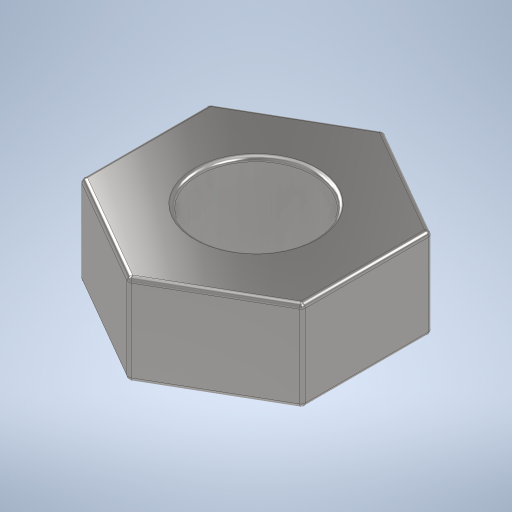
# Autodesk Inventor part: Threaded Rod Nut
Saved by Autodesk Inventor 2024 (Build 280153000, 153)
## iProperties
Created: 2023-12-05
Part Number: Threaded Rod Nut
Material: Steel, Mild
Document SubType Name: Modeling
Designer: 18179
Density: 7.85 g/cm^3
Appearance: Semi-Polished
Author: 18179
Autodesk Inventor part; units mm, degrees
ref_plane "YZ Plane" through (0, 0, 0) normal (1, 0, 0) x (0, 1, 0)
ref_plane "XZ Plane" through (0, 0, 0) normal (0, 1, 0) x (-1, 0, 0)
ref_plane "XY Plane" through (0, 0, 0) normal (0, 0, 1) x (1, 0, 0)
sketch "Sketch1" plane through (0, 0, 0) normal (0, 1, 0) x (-1, 0, 0)
  line L0 (6.75, -3.8971) -> (0, -7.7942)
  line L1 (0, -7.7942) -> (-6.75, -3.8971)
  line L2 (-6.75, -3.8971) -> (-6.75, 3.8971)
  line L3 (-6.75, 3.8971) -> (0, 7.7942)
  line L4 (0, 7.7942) -> (6.75, 3.8971)
  line L5 (6.75, 3.8971) -> (6.75, -3.8971)
  circle A0 centre (0, 0) radius 3.5
  point P0 (-6.75, 0)
  point P1 (6.75, 0)
  dimension "d0" = 13.5
  dimension "d1" = 7
  constraints: 12 end point, 2 coincident, 2 midpoint, 1 centre point, 13 other
  measures "d0" distance of point (-6.75, 0) point (6.75, 0)
  measures "d1" diameter of A0
extrude "Extrusion1" add sketch "Sketch1" along normal blind 5.5
fillet "Fillet1" radius 0.254 20 edges at (3.375, 5.5, 5.8457) (-3.375, 5.5, 5.8457) (-6.75, 5.5, 0) (-3.375, 5.5, -5.8457) (3.375, 5.5, -5.8457) (6.75, 5.5, 0) (3.5, 5.5, 0) (3.5, 0, 0) (3.375, 0, 5.8457) (6.75, 0, 0) (3.375, 0, -5.8457) (-3.375, 0, -5.8457) (-6.75, 0, 0) (-3.375, 0, 5.8457) (6.75, 2.75, 3.8971) (6.75, 2.75, -3.8971) (0, 2.75, -7.7942) (-6.75, 2.75, -3.8971) (-6.75, 2.75, 3.8971) (0, 2.75, 7.7942)
body "Solid1"
